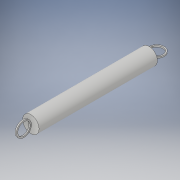
# Autodesk Inventor part: spring stand in
Saved by Autodesk Inventor 2018 (Build 220112000, 112)
## iProperties
Created: 2019-03-01
Part Number: spring stand in
Material: Generic
Document SubType Name: Modeling
Designer: s-2513225
Density: 1 g/cm^3
Appearance: Default
Author: s-2513225
Autodesk Inventor part; units mm, degrees
ref_plane "YZ Plane" through (0, 0, 0) normal (1, 0, 0) x (0, 1, 0)
ref_plane "XZ Plane" through (0, 0, 0) normal (0, 1, 0) x (-1, 0, 0)
ref_plane "XY Plane" through (0, 0, 0) normal (0, 0, 1) x (1, 0, 0)
sketch "Sketch2" plane through (0, 0, 0) normal (0, 0, 1) x (1, 0, 0)
  circle A0 centre (0, 0) radius 6.35
  dimension "d0" = 12.7
  constraints: 1 centre point, 1 coincident
  measures "d0" diameter of A0
extrude "Extrusion1" add sketch "Sketch2" along normal blind 91.059
sketch "Sketch3" plane through (0, 0, 0) normal (1, 0, 0) x (0, 1, 0)
  line L0 (6.35, 91.059) -> (-6.35, 91.059) construction
  line L1 (0, 91.059) -> (0, 96.8693) construction
  circle A0 centre (0, 96.8693) radius 5.8103
  circle A1 centre (0, 96.8693) radius 4.7943
  point P0 (0, 0)
  dimension "d3" = 5.8102
  dimension "d4" = 11.6205
  dimension "d5" = 1.016
  constraints: 2 centre point, 2 end point, 1 coincident, 1 midpoint, 1 vertical
  measures "d3" distance of L1.start L1.end
  measures "d4" diameter of A0
  measures "d5" radial gap between concentric circles of A0 A1
extrude "Extrusion2" add sketch "Sketch3" along normal mid plane 1.016
sketch "Sketch4" plane through (0, 0, 0) normal (0, 1, 0) x (-1, 0, 0)
  line L0 (0, 0) -> (0, -5.8102) construction
  circle A0 centre (0, -5.8102) radius 5.8102
  circle A1 centre (0, -5.8102) radius 4.7942
  dimension "d8" = 5.8102
  dimension "d9" = 11.6205
  dimension "d10" = 1.016
  constraints: 2 centre point, 2 end point, 1 coincident, 1 vertical
  measures "d8" distance of L0.start L0.end
  measures "d9" diameter of A0
  measures "d10" radial gap between concentric circles of A0 A1
extrude "Extrusion3" add sketch "Sketch4" along normal mid plane 1.016
body "Solid1"
